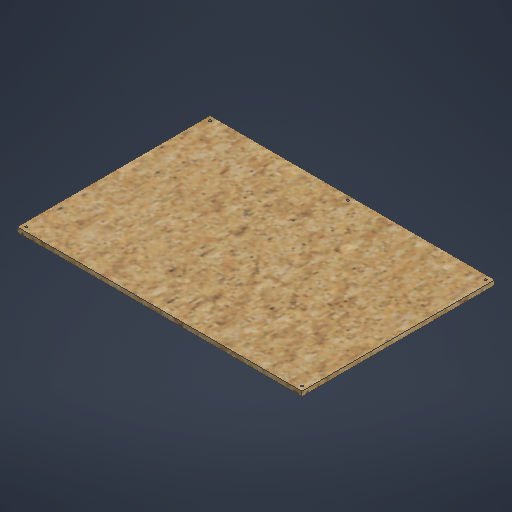
# Autodesk Inventor part: CaraLateral
Saved by Autodesk Inventor 2026.2 (Build 302298010, 298A)
## iProperties
Created: 2026-04-15
Part Number: CaraLateral
Material: Generic
Document SubType Name: Modeling
Designer: grego
Density: 1 g/cm^3
Appearance: Default
Author: grego
Autodesk Inventor part; units mm, degrees
ref_plane "YZ Plane" through (0, 0, 0) normal (1, 0, 0) x (0, 1, 0)
ref_plane "XZ Plane" through (0, 0, 0) normal (0, 1, 0) x (-1, 0, 0)
ref_plane "XY Plane" through (0, 0, 0) normal (0, 0, 1) x (1, 0, 0)
sketch "Sketch1" plane through (0, 0, 0) normal (0, 1, 0) x (-1, 0, 0)
  line L0 (-310, 210) -> (310, 210)
  line L1 (310, 210) -> (310, -210)
  line L2 (310, -210) -> (-310, -210)
  line L3 (-310, -210) -> (-310, 210)
  line L4 (-300, -200) -> (300, -200)
  line L5 (300, -200) -> (300, 200)
  line L6 (300, 200) -> (-300, 200)
  line L7 (-300, 200) -> (-300, -200)
  circle A0 centre (300, -200) radius 2.5
  circle A1 centre (-300, -200) radius 2.5
  circle A2 centre (0, -200) radius 2.5
  circle A3 centre (300, 200) radius 2.5
  circle A4 centre (-300, 200) radius 2.5
  point P0 (0, 0)
  dimension "d0" = 620
  dimension "d1" = 420
  dimension "d2" = 10
  dimension "d3" = 5
  dimension "d4" = 5
  dimension "d5" = 5
  dimension "d6" = 5
  dimension "d7" = 5
  constraints: 16 end point, 5 centre point, 4 coincident, 4 parallel, 2 perpendicular, 1 horizontal, 1 midpoint, 3 other
  measures "d0" distance of L1.end L2.end
  measures "d1" distance of L0.end L1.end
  measures "d2" distance between parallel lines of L2 L4
  measures "d3" diameter of A0
  measures "d4" diameter of A1
  measures "d5" diameter of A2
  measures "d6" diameter of A3
  measures "d7" diameter of A4
extrude "Extrusion1" add sketch "Sketch1" along normal blind 10 contours L0 L1 L2 L3 | A1 L7 A4 L6 A3 L5 A0 L4 A2
body "Solid1"
